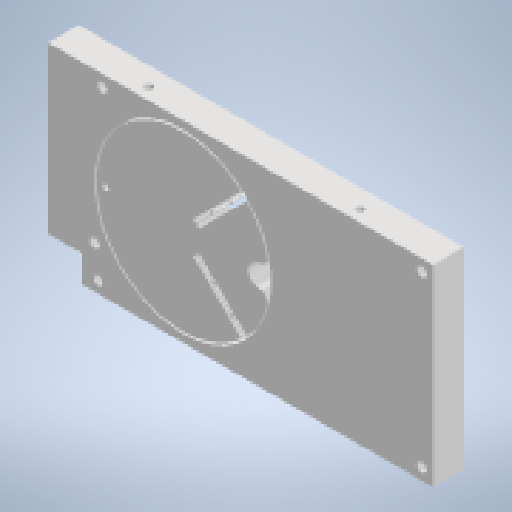
# Autodesk Inventor part: RoueV3partA
Saved by Autodesk Inventor 2023 (Build 270158000, 158)
## iProperties
Created: 2023-04-29
Part Number: RoueV3partA
Material: Generic
Document SubType Name: Modeling
Designer: Nathann
Density: 1 g/cm^3
Appearance: Default
Author: Nathann
Autodesk Inventor part; units mm, degrees
ref_plane "YZ Plane" through (0, 0, 0) normal (1, 0, 0) x (0, 1, 0)
ref_plane "XZ Plane" through (0, 0, 0) normal (0, 1, 0) x (-1, 0, 0)
ref_plane "XY Plane" through (0, 0, 0) normal (0, 0, 1) x (1, 0, 0)
sketch "Sketch1" plane through (0, 0, 0) normal (0, 0, 1) x (1, 0, 0)
  line L0 (0, 0) -> (100, 0)
  line L1 (100, 0) -> (100, 50)
  line L2 (100, 50) -> (0, 50)
  line L3 (0, 50) -> (0, 0)
  circle A0 centre (95, 45) radius 1.75
  circle A1 centre (95, 5) radius 1.75
  circle A2 centre (15, 45) radius 1.75
  circle A3 centre (15, 5) radius 1.75
  dimension "d0" = 50
  dimension "d1" = 100
  dimension "d2" = 5
  dimension "d3" = 5
  dimension "d4" = 5
  dimension "d5" = 5
  dimension "d6" = 5
  dimension "d7" = 15
  dimension "d8" = 15
  dimension "d9" = 5
  dimension "d10" = 3.5
  dimension "d11" = 3.5
  dimension "d12" = 3.5
  dimension "d13" = 3.5
  constraints: 8 end point, 4 centre point, 2 parallel, 1 horizontal, 1 perpendicular
  measures "d0" distance of L2.end L0.start
  measures "d1" distance of L1.end L2.end
  measures "d2" distance from line of L1 A0.centre
  measures "d3" distance from line of A0.centre L2
  measures "d4" distance from line of L0 A1.centre
  measures "d5" distance from line of L1 A1.centre
  measures "d6" distance from line of L2 A2.centre
  measures "d7" distance from line of A2.centre L3
  measures "d8" distance from line of L3 A3.centre
  measures "d9" distance from line of L0 A3.centre
  measures "d10" diameter of A3
  measures "d11" diameter of A0
  measures "d12" diameter of A2
  measures "d13" diameter of A1
extrude "Extrusion1" add sketch "Sketch1" along normal blind 8 contours L3 L2 L1 L0 | A0 | A1 | A2 | A3
sketch "Sketch4" plane through (0, 0, 8) normal (0, 0, 1) x (1, 0, 0)
  circle A0 centre (15, 25) radius 0.8
  circle A1 centre (55, 25) radius 3
  line L0 (0, 50) -> (0, 0) projected
  line L1 (35, 25) -> (52.9141, 42.9141)
  line L2 (35, 25) -> (41.4896, 25)
  line L3 (35, 25) -> (55.1987, 4.8013)
  circle A2 centre (35, 25) radius 23
  line L4 (0, 0) -> (100, 0) projected
  circle A3 centre (35, 25) radius 5
  line L5 (38.5, 28.5707) -> (51.2281, 41.2988)
  line L6 (37.757, 29.1712) -> (50.1871, 41.6013)
  line L7 (38.5707, 28.5) -> (51.2988, 41.2281)
  line L8 (51.6013, 40.1871) -> (39.1712, 27.757)
  line L9 (38.5707, 21.5) -> (51.2988, 8.7719)
  line L10 (38.5, 21.4293) -> (51.2281, 8.7012)
  line L11 (37.757, 20.8288) -> (50.1871, 8.3987)
  line L12 (39.1712, 22.243) -> (51.6013, 9.8129)
  arc A4 (51.6013, 9.8129) -> (50.1871, 8.3987) centre (35, 25) ccw
  circle A5 centre (41.2925, 32.7067) radius 0.95
  circle A6 centre (42.7067, 34.121) radius 0.95
  circle A7 centre (46.2423, 37.6565) radius 0.95
  circle A8 centre (47.6565, 39.0707) radius 0.95
  circle A9 centre (42.7067, 18.7075) radius 0.95
  circle A10 centre (44.121, 17.2933) radius 0.95
  circle A11 centre (47.6565, 13.7577) radius 0.95
  circle A12 centre (49.0707, 12.3435) radius 0.95
  point P0 (0, 15)
  point P1 (7, 0)
  point P2 (57.4312, 26.7576)
  point P3 (57.4312, 23.2424)
  point P4 (58, 25)
  point P5 (50.9452, 40.8745)
  point P6 (50.8745, 40.9452)
  point P7 (41.9643, 32.035)
  point P8 (41.9643, 33.3785)
  point P9 (42.035, 33.4492)
  point P10 (43.3785, 33.4492)
  point P11 (46.914, 36.9847)
  point P12 (46.914, 38.3282)
  point P13 (48.3282, 38.399)
  point P14 (46.9847, 38.399)
  point P15 (42.035, 18.0357)
  point P16 (43.3785, 18.0357)
  point P17 (43.4492, 17.965)
  point P18 (43.4492, 16.6215)
  point P19 (46.9847, 13.086)
  point P20 (48.3282, 13.086)
  point P21 (48.399, 13.0153)
  point P22 (48.399, 11.6718)
  dimension "d34" = 10
  dimension "d22" = 15
  dimension "d23" = 40
  dimension "d24" = 20
  dimension "d26" = 1.6
  dimension "d27" = 6
  dimension "d28" = 45
  dimension "d29" = 45
  dimension "d30" = 46
  dimension "d31" = 25
  dimension "d32" = 25
  dimension "d33" = 25
  dimension "d35" = 1
  dimension "d36" = 1
  dimension "d37" = 0.1
  dimension "d38" = 0.05
  dimension "d39" = 0.1
  dimension "d40" = 0.05
  dimension "d41" = 1
  dimension "d42" = 1
  dimension "d79" = 5
  dimension "d80" = 2
  dimension "d81" = 5
  dimension "d82" = 2
  dimension "d83" = 5
  dimension "d84" = 2
  dimension "d85" = 5
  dimension "d86" = 2
  constraints: 22 end point, 12 centre point, 8 point on circle, 8 point on line, 8 tangent, 7 parallel, 2 coincident, 1 horizontal, 10 other
  measures "d22" distance from line of L0 A0.centre
  measures "d23" distance of A1.centre A0.centre
  measures "d24" distance of A1.centre L1.start
  measures "d26" diameter of A0
  measures "d27" diameter of A1
  measures "d28" angle of L3 L2
  measures "d29" angle of L1 L2
  measures "d30" diameter of A2
  measures "d31" distance from line of L4 L1.start
  measures "d32" distance from line of L4 A0.centre
  measures "d33" distance from line of L4 A1.centre
  measures "d35" distance between parallel lines of L6 L1
  measures "d36" distance between parallel lines of L8 L1
  measures "d37" distance between parallel lines of L7 L5
  measures "d38" distance between parallel lines of L1 L5
  measures "d39" distance between parallel lines of L9 L10
  measures "d40" distance between parallel lines of L3 L10
  measures "d41" distance between parallel lines of L12 L3
  measures "d42" distance between parallel lines of L11 L3
  measures "d79" distance of A5.centre L6.start
  measures "d80" distance of A6.centre A5.centre
  measures "d81" distance of A7.centre A6.centre
  measures "d82" distance of A8.centre A7.centre
  measures "d83" distance of A9.centre L12.start
  measures "d84" distance of A9.centre A10.centre
  measures "d85" distance of A10.centre A11.centre
  measures "d86" distance of A12.centre A11.centre
extrude "Extrusion4" cut sketch "Sketch4" against normal blind 8 contours A0 | A1 A4 | A2 L9 A12 L12 A4 A1 | A1 A4 L7 A2 | A4 A1 | L8 A3 L7 A4 | A12 L12 | L5 A4 L11 A3 L10 A2 | L9 A10 L12 A11 | A11 L12 | L5 A8 L6 A4 | A3 L12 A9 L9 | A10 L12 | A3 L6 A5 L5 | A8 L6 | A9 L12 | A5 L6 | L5 A6 L6 A7 | A7 L6 | A6 L6 picked at (49.0352, 12.0288) picked at (47.3576, 13.4145) picked at (44.1564, 16.9786) picked at (47.9671, 39.0089) picked at (42.6021, 18.4086) picked at (41.6092, 32.7067) picked at (46.2068, 37.3418) picked at (43.0173, 33.7349)
fillet "Fillet2" radius 2 2 edges at (57.4312, 26.7576, 4) (57.4312, 23.2424, 4)
sketch "Sketch5" plane through (0, 0, 0) normal (-1, 0, 0) x (0, 0, 1)
  line L0 (0, 0) -> (1.5, 0)
  line L1 (1.5, 0) -> (1.5, 15)
  line L2 (1.5, 15) -> (0, 15)
  line L3 (0, 15) -> (0, 0)
  line L4 (8, 0) -> (8, 50) projected
  line L5 (8, 0) -> (1.5, 0)
  line L6 (1.5, 0) -> (1.5, 7)
  line L7 (1.5, 7) -> (8, 7)
  line L8 (8, 7) -> (8, 0)
  dimension "d47" = 15
  dimension "d48" = 1.5
  dimension "d51" = 7
  constraints: 16 end point, 4 parallel, 2 horizontal, 2 perpendicular, 1 point on line
  measures "d47" distance of L0.end L1.end
  measures "d48" distance of L1.end L2.end
  measures "d51" distance between parallel lines of L5 L7
extrude "Extrusion5" cut sketch "Sketch5" against normal blind 9
sketch "Sketch6" plane through (0, 7, 1.5) normal (0, -1, 0) x (1, 0, 0)
  circle A0 centre (6.75, 1.2764) radius 1.1 projected
  circle A1 centre (1.25, 1.2764) radius 1.1 projected
  circle A2 centre (6.75, 1.2764) radius 0.8
  circle A3 centre (1.25, 1.2764) radius 0.8
  point P0 (0, -1.5)
  dimension "d52" = 1.6
  dimension "d53" = 1.6
  constraints: 2 centre point, 2 coincident
  measures "d52" diameter of A2
  measures "d53" diameter of A3
extrude "Extrusion6" cut sketch "Sketch6" against normal blind 8 contours A2 | A3
sketch "Sketch7" plane through (0, 0, 8) normal (0, 0, 1) x (1, 0, 0)
  circle A0 centre (97, 3) radius 1.7 projected
  circle A1 centre (97, 47) radius 1.7 projected
  circle A2 centre (12, 11) radius 1.7 projected
  circle A3 centre (21.5, 47.5) radius 1.7 projected
  circle A4 centre (97, 3) radius 1.25
  circle A5 centre (97, 47) radius 1.25
  circle A6 centre (13, 3) radius 1.25
  circle A7 centre (12, 11) radius 1.25
  circle A8 centre (21.5, 47.5) radius 1.25
  circle A9 centre (14, 47) radius 1.7
  circle A10 centre (14, 47) radius 1.25
  line L0 (9, 0) -> (100, 0) projected
  line L1 (9, 0) -> (9, 15) projected
  point P0 (0, 0)
  dimension "d56" = 2.5
  dimension "d57" = 2.5
  dimension "d58" = 2.5
  dimension "d59" = 2.5
  dimension "d60" = 2.5
  dimension "d63" = 2.5
  dimension "d64" = 3
  dimension "d65" = 4
  constraints: 7 centre point, 5 coincident, 2 other
  measures "d56" diameter of A4
  measures "d57" diameter of A5
  measures "d58" diameter of A6
  measures "d59" diameter of A7
  measures "d60" diameter of A8
  measures "d63" diameter of A10
  measures "d64" distance from line of L0 A6.centre
  measures "d65" distance from line of L1 A6.centre
extrude "Extrusion7" cut sketch "Sketch7" against normal blind 8 contours A4 | A5 | A6 | A7 | A10
sketch "Sketch8" plane through (0, 50, 0) normal (0, 1, 0) x (1, 0, 0)
  circle A0 centre (23, -5) radius 1.375
  circle A1 centre (78, -5) radius 1.375
  circle A2 centre (23, -5) radius 1.025
  circle A3 centre (78, -5) radius 1.025
  line L0 (0, 0) -> (0, -8) projected
  dimension "d68" = 2.05
  dimension "d69" = 2.05
  dimension "d74" = 23
  dimension "d75" = 23
  dimension "d76" = 55
  constraints: 4 centre point, 1 coincident
  measures "d68" diameter of A3
  measures "d69" diameter of A2
  measures "d74" distance from line of A0.centre L0
  measures "d75" distance from line of L0 A2.centre
  measures "d76" distance of A1.centre A0.centre
extrude "Extrusion8" cut sketch "Sketch8" against normal blind 8 contours A2 | A3
sketch "Sketch9" plane through (100, 0, 0) normal (0, -1, 0) x (1, 0, 0)
  circle A0 centre (-77, 5) radius 1.375
  circle A1 centre (-22, 5) radius 1.375
  circle A2 centre (-77, 5) radius 1.025
  circle A3 centre (-22, 5) radius 1.025
  line L0 (-100, 1.5) -> (-100, 8) projected
  point P0 (-100, 0)
  dimension "d70" = 2.05
  dimension "d71" = 2.05
  dimension "d77" = 23
  dimension "d78" = 55
  constraints: 4 centre point, 2 coincident
  measures "d70" diameter of A2
  measures "d71" diameter of A3
  measures "d77" distance from line of A0.centre L0
  measures "d78" distance of A1.centre A0.centre
extrude "Extrusion9" cut sketch "Sketch9" against normal blind 8 contours A2 | A3
equation "\"d4\" = d3"
equation "\"d5\" = d2"
equation "\"d6\" = d3"
equation "\"d9\" = d4"
equation "\"d10\" = d11"
equation "\"d12\" = d11"
equation "\"d13\" = d11"
equation "\"d24\" = 0.5 * d23"
equation "\"d37\" = BladeThicknessRCC"
equation "\"d38\" = 0.5 * d37"
equation "\"d39\" = BladeThicknessRCC"
equation "\"d40\" = 0.5 * BladeThicknessRCC"
equation "\"d59\" = d58"
equation "\"d60\" = d59"
equation "\"d75\" = d74"
equation "\"bladeThicknessTablePushing\" = 0.1"
equation "\"bladeThicknessTable\" = 0.1"
equation "\"bladeThicknessForceConverter\" = 0.2"
equation "\"bladeThicknessWheelAnchor\" = 0.1"
equation "\"safetyPlay\" = 0.1"
equation "\"OffsetMotorSpring\" = -1"
equation "\"BladeThicknessRCC\" = 0.1"
equation "\"bladeThicknessZeroConverter\" = 0.1"
equation "\"rangeXProbeMin\" = -0.6"
equation "\"thicknessWheelPlate\" = 8"
equation "\"rangeXProbeMax\" = 0.6"
equation "\"BladeLengthRCC\" = 18"
equation "\"bladeLengthTable\" = 18"
equation "\"bladeLengthWheelAnchor\" = 7.5"
equation "\"RCCdeadCenter\" = 5"
equation "\"bladeLengthZeroConverter\" = 11.98"
equation "\"bladeLengthTablePushing\" = 12"
equation "\"bladeLengthForceConverter\" = 12.125"
equation "\"thicknessConverterPlate\" = 4"
body "Solid1"
